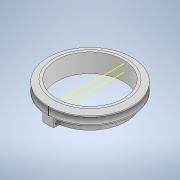
# Autodesk Inventor part: adapter_za_motor
Saved by Autodesk Inventor 2021 (Build 250183000, 183)
## iProperties
Created: 2024-10-27
Part Number: adapter_za_motor
Material: Generic
Document SubType Name: Modeling
Designer: Ben
Density: 1 g/cm^3
Appearance: Default
Author: Ben
Autodesk Inventor part; units mm, degrees
ref_plane "YZ Plane" through (0, 0, 0) normal (1, 0, 0) x (0, 1, 0)
sketch "Sketch1" plane through (0, 0, 0) normal (0, 0, 1) x (1, 0, 0)
  line L0 (0, 0) -> (-171.0711, 0) construction
  line L1 (0, 0) -> (0, -629.6601) construction
  line L2 (-62.5, 0) -> (-62.5, -35)
  line L3 (-62.5, -35) -> (-67.5, -35)
  line L4 (-62.5, 0) -> (-67.5, 0)
  line L5 (-67.5, 0) -> (-78.5, -4.0037)
  line L6 (-78.5, -4.0037) -> (-78.5, -6.0037)
  line L7 (-78.5, -6.0037) -> (-67.5, -10.0073)
  line L8 (-67.5, -10.0073) -> (-67.5, -14.0073)
  line L9 (-67.5, -14.0073) -> (-78.5, -18.011)
  line L10 (-78.5, -18.011) -> (-78.5, -20.011)
  line L11 (-67.5, -35) -> (-67.5, 0) construction
  line L12 (-78.5, -20.011) -> (-67.5, -24.0147)
  line L13 (-78.5, -20.011) -> (-66.794, -20.011) construction
  line L14 (-67.5, -24.0147) -> (-67.5, -35)
  line L15 (-62.5, -33.4145) -> (-62.8994, -35)
  dimension "d1" = 35
  dimension "d2" = 5
  dimension "d3" = 5
  dimension "d6" = 2
  dimension "d8" = 2
  dimension "d10" = 40
  dimension "d11" = 62.5
  dimension "d12" = 20
  dimension "d13" = 4
  dimension "d14" = 11
  dimension "d15" = 5
  constraints: 32 end point, 5 point on line, 4 parallel, 3 vertical, 2 collinear, 2 horizontal, 1 equal length, 1 perpendicular
  measures "d1" distance of L2.start L2.end
  measures "d2" distance of L2.end L3.end
  measures "d3" distance of L2.start L4.end
  measures "d6" distance of L5.end L6.end
  measures "d8" distance of L9.end L10.end
  measures "d10" angle of L9 L7
  measures "d11" distance between parallel lines of L1 L2
  measures "d12" angle of L0 L5
  measures "d13" distance of L7.end L8.end
  measures "d14" distance between parallel lines of L8 L6
  measures "d15" distance between parallel lines of L2 L8
revolve "Revolution1" add sketch "Sketch1" angle 360 about axis through (0, 0, 0) along (0, -1, 0)
sketch "Sketch2" plane through (0, 0, 0) normal (0, 0, 1) x (1, 0, 0)
  point P0 (0, 0)
sketch "Sketch3" plane through (0, 0, 0) normal (1, 0, 0) x (0, 1, 0)
  line L0 (-6.0037, -78.5) -> (-4.0037, -78.5) projected
  line L1 (-20.011, -78.5) -> (-18.011, -78.5) projected
  line L2 (-4.0037, -78.5) -> (-20.011, -78.5)
  line L3 (-6.0037, -78.5) -> (-6.0037, 78.5) projected
  line L4 (-6.0037, 78.5) -> (-4.0037, 78.5) projected
  line L5 (-20.011, 78.5) -> (-18.011, 78.5) projected
  line L6 (-20.011, -78.5) -> (-20.011, 78.5) projected
  line L7 (-20.011, 78.5) -> (-4.0037, 78.5)
  point P0 (0, 0)
  constraints: 4 end point, 2 perpendicular
ref_plane "Work Plane1" through (0, -4.0037, -78.5) normal (0, 0, -1) x (-1, 0, 0)
sketch "Sketch4" plane through (0, -4.0037, -78.5) normal (0, 0, -1) x (-1, 0, 0)
  line L0 (67.5, -30.9963) -> (-67.5, -30.9963) projected
  line L1 (10, -30.9963) -> (-10, -30.9963)
  line L2 (-10, -30.9963) -> (-10, -16.0073)
  line L3 (-10, -16.0073) -> (10, -16.0073)
  line L4 (10, -16.0073) -> (10, -30.9963)
  line L5 (0, 0) -> (0, -16.0073) projected
  point P0 (0, 4.0037)
  dimension "d17" = 20
  dimension "d18" = 10
  constraints: 8 end point, 2 parallel, 2 point on line, 1 perpendicular
  measures "d17" distance between parallel lines of L4 L2
  measures "d18" distance between parallel lines of L4 L5
ref_plane "Work Plane2" through (0, -20.011, 78.5) normal (0, 0, 1) x (1, 0, 0)
extrude "Extrusion1" add sketch "Sketch4" against normal up to surface (157 mm away)
sketch "Sketch5" plane through (0, -20.011, 0) normal (0, 1, 0) x (1, 0, 0)
  circle A0 centre (0, 0) radius 62.5 projected
  arc A1 (-10, -61.6948) -> (10, -61.6948) centre (0, 0) ccw projected
  line L0 (10, 61.6948) -> (10, -61.6948) projected
  arc A2 (10, 61.6948) -> (-10, 61.6948) centre (0, 0) ccw projected
  line L1 (-10, 61.6948) -> (-10, -61.6948) projected
  arc A3 (-10, -77.8605) -> (0, -78.5) centre (0, 0) ccw projected
  line L2 (-10, -77.8605) -> (-10, -78.5) projected
  line L3 (-10, -78.5) -> (0, -78.5) projected
  arc A4 (0, -78.5) -> (10, -77.8605) centre (0, 0) ccw projected
  line L4 (0, -78.5) -> (10, -78.5) projected
  line L5 (10, -77.8605) -> (10, -78.5) projected
  arc A5 (0, 78.5) -> (-10, 77.8605) centre (0, 0) ccw projected
  line L6 (-10, 78.5) -> (0, 78.5) projected
  line L7 (-10, 78.5) -> (-10, 77.8605) projected
  arc A6 (10, 77.8605) -> (0, 78.5) centre (0, 0) ccw projected
  line L8 (10, 78.5) -> (10, 77.8605) projected
  line L9 (0, 78.5) -> (10, 78.5) projected
  point P0 (0, -78.5)
  point P1 (0, -78.5)
  point P2 (0, -78.5)
  point P3 (0, -78.5)
  point P4 (-10, 61.6948)
  point P5 (-10, -61.6948)
  point P6 (10, -61.6948)
extrude "Extrusion2" cut sketch "Sketch5" against normal through all contours L0 A0 L1 | A4 L5 L4 | A3 L3 L2 | A5 L7 L6 | L9 L8 A6
sketch "Sketch6" plane through (10, -35, -77.8605) normal (1, 0, 0) x (0, 0, -1)
  line L0 (0, 0) -> (0.6395, 0) construction
  line L1 (-11.1053, 10.9853) -> (-11.1053, 0) construction
  line L2 (0.6395, 0) -> (-11.1053, 10.9853) construction
  circle A0 centre (-5.2329, 5.4927) radius 3
  line L3 (-144.6156, 10.9853) -> (-144.6156, 0) construction
  line L4 (-155.7209, 14.989) -> (-155.7209, 0) construction
  line L5 (-144.6156, 10.9853) -> (-155.7209, 0) construction
  circle A1 centre (-150.1683, 5.4927) radius 3
  point P0 (-77.8605, 35)
  dimension "d23" = 6
  dimension "d24" = 6
  constraints: 4 end point, 2 centre point, 2 midpoint
  measures "d23" diameter of A0
  measures "d24" diameter of A1
extrude "Extrusion3" cut sketch "Sketch6" against normal through all
body "Solid1"
